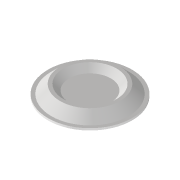
# Autodesk Inventor part: 50_ETL_Membrane_v0
Saved by Autodesk Inventor 2022 (Build 260153000, 153)
## iProperties
Created: 2021-12-31
Part Number: 50_ETL_Membrane_v0
Material: Generisch
Document SubType Name: Modeling
Designer: diederichbenedict
Density: 1 g/cm^3
Appearance: Vorgabe
Author: diederichbenedict
Autodesk Inventor part; units mm, degrees
ref_plane "YZ Plane" through (0, 0, 0) normal (1, 0, 0) x (0, 1, 0)
ref_plane "XZ Plane" through (0, 0, 0) normal (0, 1, 0) x (-1, 0, 0)
ref_plane "XY Plane" through (0, 0, 0) normal (0, 0, 1) x (1, 0, 0)
sketch "Skizze1" plane through (0, 0, 0) normal (1, 0, 0) x (0, 1, 0)
  line L0 (3, 8.0893) -> (5.1212, 8.0893) construction
  line L1 (-0.0509, -6.2) -> (0.0741, -6.2) construction
  line L2 (0.0741, -6.2) -> (0.0741, 6.2) construction
  line L3 (0.0741, 6.2) -> (-0.0509, 6.2) construction
  line L4 (-0.0509, 6.2) -> (-0.0509, -6.2) construction
  line L5 (-0.0509, -6.2) -> (0.0741, 6.2) construction
  line L6 (0.0741, -6.2) -> (-0.0509, 6.2) construction
  line L7 (-0.0509, 6.2) -> (-0.0509, 0)
  line L8 (-0.0509, 0) -> (-0.7509, 0)
  line L9 (-0.7509, 0) -> (-0.7509, 7.0138)
  line L10 (-0.7509, 7.0138) -> (0.4491, 8.2138)
  line L11 (0.4491, 8.2138) -> (0.4491, 8.4858)
  line L12 (-0.0509, 6.2) -> (-0.0509, 6.4)
  line L13 (-0.0509, 6.4) -> (1.4491, 7.9)
  line L14 (1.4491, 7.9) -> (1.4491, 8.9)
  line L15 (1.4491, 8.9) -> (-1.1509, 11.5)
  line L16 (-1.7509, 12.5) -> (-1.7509, 9.4858)
  line L17 (0.4491, 8.4858) -> (-0.5509, 9.4858)
  line L18 (-0.5509, 9.4858) -> (-1.7509, 9.4858)
  line L19 (-1.1509, 11.5) -> (-1.1509, 12.5)
  line L20 (-1.1509, 12.5) -> (-1.7509, 12.5)
  line L21 (1.4491, 8.9) -> (1.4491, -8.9) projected
  line L22 (-1.1509, 11.5) -> (1.4491, 8.9)
  line L23 (1.4491, 7.9) -> (0.1491, 6.6)
  point P0 (0.0116, 0)
  point P1 (0.0116, 0)
  dimension "d14" = 0.125
  dimension "d16" = 0.7
  dimension "d18" = 135
  dimension "d20" = 0.2
  dimension "d27" = 135
  dimension "d28" = 1
  dimension "d29" = 1.2
  dimension "d30" = 1
  dimension "d31" = 1
  dimension "d34" = 1
  dimension "d36" = 0.6
  dimension "d37" = 12.5
  dimension "d39" = 1
  constraints: 46 end point, 5 midpoint, 4 horizontal, 4 parallel, 4 perpendicular, 3 vertical, 1 point on line, 5 other
  measures "d14" distance of L3.end L2.end
  measures "d16" distance of L7.end L8.end
  measures "d18" angle of L9 L10
  measures "d20" distance of L3.end L12.end
  measures "d27" angle of L11 L17
  measures "d28" distance from line of L17.end L11
  measures "d29" distance between parallel lines of L9 L11
  measures "d30" distance between parallel lines of L11 L14
  measures "d31" distance between parallel lines of L15 L17
  measures "d34" distance between parallel lines of L9 L16
  measures "d36" distance between parallel lines of L19 L16
  measures "d37" distance between parallel lines of L8 L20
  measures "d39" distance from line of L15.end L20
revolve "Umdrehung1" add sketch "Skizze1" angle 360 about axis through (0, -0.0509, 0) along (0, -1, 0)
